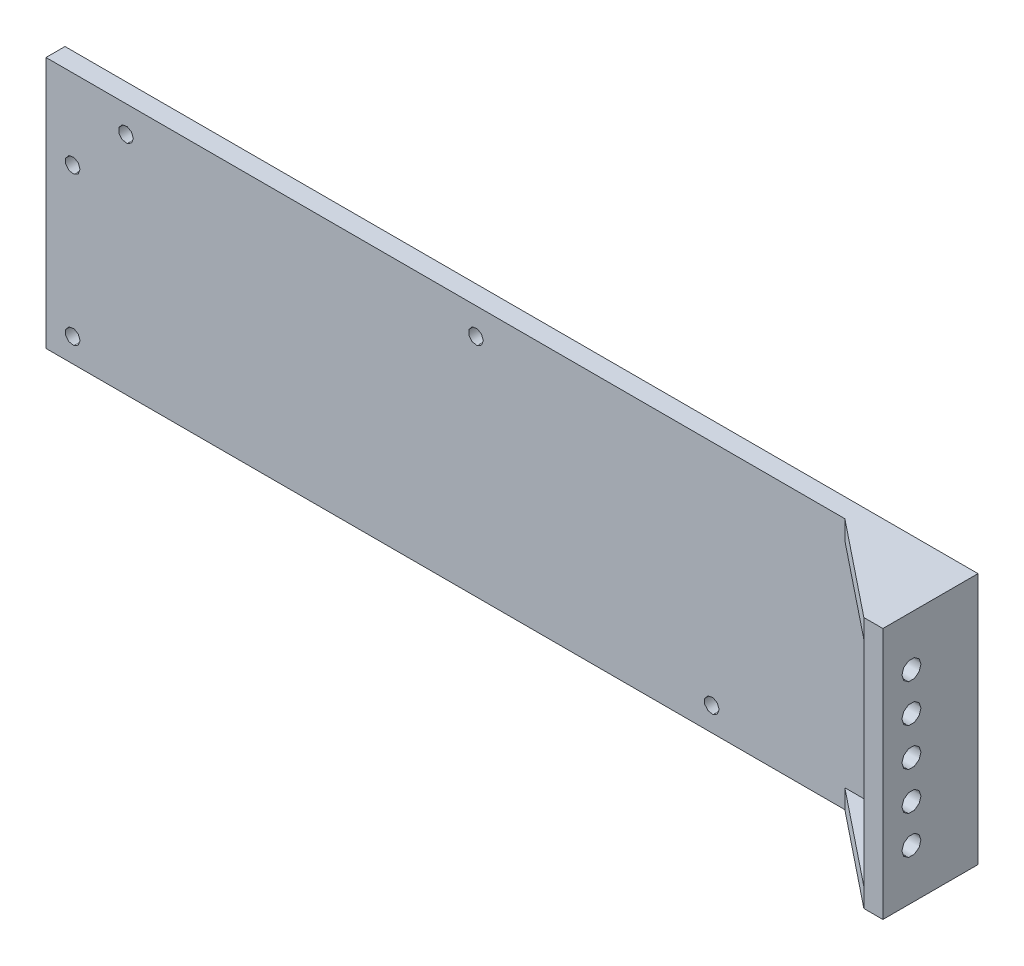
# Autodesk Inventor part: dilution system bracket
Saved by Autodesk Inventor 2022 (Build 260153000, 153)
## iProperties
Created: 2021-12-08
Part Number: dilution system bracket
Material: Generic
Document SubType Name: Modeling
Designer: efred
Density: 1 g/cm^3
Appearance: Default
Author: efred
Autodesk Inventor part; units mm, degrees
ref_plane "YZ Plane" through (0, 0, 0) normal (1, 0, 0) x (0, 1, 0)
ref_plane "XZ Plane" through (0, 0, 0) normal (0, 1, 0) x (-1, 0, 0)
ref_plane "XY Plane" through (0, 0, 0) normal (0, 0, 1) x (1, 0, 0)
ref_plane "Work Plane1" through (0, 0, 0) normal (0, 0, 1) x (1, 0, 0)
sketch "Sketch1" plane through (0, 0, 0) normal (0, 0, 1) x (1, 0, 0)
  line L0 (91, 0.01) -> (-91, 0.01) construction
  line L1 (91, 0.01) -> (91, 13.01) construction
  line L2 (28.25, 66.26) -> (91, 13.01) construction
  line L3 (-75.75, 66.26) -> (28.25, 66.26) construction
  line L4 (-91, 51.01) -> (-75.75, 66.26) construction
  line L5 (-91, 0.01) -> (-91, 51.01) construction
  circle A0 centre (22, 59.26) radius 1.95 projected
  circle A1 centre (-84, 6.26) radius 1.95 projected
  circle A2 centre (-84, 45.26) radius 1.95 projected
  circle A3 centre (-70, 59.26) radius 1.95 projected
  line L6 (149.1, -0.3275) -> (149.1, 180.6725) construction
  line L7 (-91, 0.01) -> (149, 0.01)
  line L8 (149, 0.01) -> (149, 66.26)
  line L9 (149, 66.26) -> (-91, 66.26)
  line L10 (-91, 66.26) -> (-91, 0.01)
  circle A4 centre (84, 6.26) radius 1.95 projected
  point P0 (0, 0)
  dimension "d0" = 0.1
  constraints: 8 end point, 2 parallel, 1 collinear, 1 horizontal, 1 perpendicular
  measures "d0" distance between parallel lines of L6 L8
extrude "Extrusion1" add sketch "Sketch1" along normal blind 5
sketch "Sketch2" plane through (0, 0, 5) normal (0, 0, 1) x (1, 0, 0)
  line L0 (149, 0.01) -> (149, 66.26) projected
  line L1 (149, 66.26) -> (-91, 66.26) projected
  line L2 (149, 0.01) -> (144, 0.01)
  line L3 (144, 0.01) -> (144, 66.26)
  line L4 (144, 66.26) -> (149, 66.26)
  line L5 (149, 66.26) -> (149, 0.01)
  point P0 (0, 0)
  dimension "d3" = 5
  constraints: 8 end point, 2 parallel, 1 horizontal, 1 perpendicular, 1 point on line
  measures "d3" distance between parallel lines of L0 L3
extrude "Extrusion2" add sketch "Sketch2" along normal blind 20
fillet "Fillet1" radius 5 1 edges at (144, 33.135, 5)
sketch "Sketch3" plane through (-91, 66.26, 0) normal (0, 1, 0) x (1, 0, 0)
  line L0 (240, -25) -> (235, -25) projected
  line L1 (235, -25) -> (210, -5)
  line L2 (230, -5) -> (0, -5) projected
  line L3 (235, -10) -> (235, -25) projected
  arc A0 (235, -10) -> (230, -5) centre (230, -10) ccw projected
  point P0 (91, 0)
  dimension "d7" = 20
  constraints: 2 end point, 1 point on line
  measures "d7" distance of L2.start L1.end
extrude "Extrusion3" add sketch "Sketch3" against normal blind 5
ref_plane "Work Plane2" through (-91, 33.135, 0) normal (0, -1, 0) x (1, 0, 0)
mirror "Mirror1" about plane through (-91, 33.135, 0) normal (0, -1, 0) of "Extrusion3"
sketch "Sketch4" plane through (144, 61.26, 10) normal (-1, 0, 0) x (0, 0, 1)
  line L0 (0, -56.25) -> (15, -56.25) projected
  line L1 (15, 0) -> (15, -56.25) projected
  line L2 (15, 0) -> (0, 0) projected
  line L3 (0, -56.25) -> (0, 0) projected
  circle A0 centre (7.5, -18.125) radius 2.5
  circle A1 centre (7.5, -38.125) radius 2.5
  circle A2 centre (7.5, -28.125) radius 2.5
  line L4 (0, -56.25) -> (0, 0) projected
  line L5 (0, -28.125) -> (15, -28.125) construction
  line L6 (15, -61.25) -> (15, 5) projected
  circle A3 centre (7.5, -8.125) radius 2.5
  circle A4 centre (7.5, -48.125) radius 2.5
  point P0 (-10, -61.26)
  point P1 (7.5, -28.125)
  dimension "d10" = 5
  dimension "d11" = 5
  dimension "d12" = 10
  dimension "d13" = 5
  dimension "d14" = 10
  constraints: 5 centre point, 3 midpoint, 2 end point, 2 vertical alignment, 1 coincident, 1 symmetric about line, 2 other
  measures "d10" diameter of A0
  measures "d11" diameter of A2
  measures "d12" distance of A2.centre A0.centre
  measures "d13" diameter of A3
  measures "d14" distance of A0.centre A3.centre
extrude "Extrusion4" cut sketch "Sketch4" against normal through all contours A0 | A1 | A2 | A3 | A4
body "Solid1"
